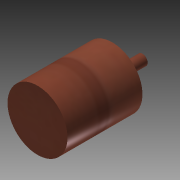
# Autodesk Inventor part: motor
Saved by Autodesk Inventor 2014 (Build 180170000, 170)
## iProperties
Created: 2014-11-30
Part Number: motor
Material: Generic
Document SubType Name: Modeling
Designer: ph1140784
Density: 1 g/cm^3
Appearance: Metal - Ribbed Copper
Mass: 63.6015 g
Surface Area: 92.3628 cm^2
Volume: 63.6015 cm^3
d0: 40.000 mm
d1: 50.000 mm
d2: 0.00 deg
d3: 7.000 mm
d4: 20.000 mm
d5: 0.00 deg
Author: ph1140784
Autodesk Inventor part; units mm, degrees
ref_plane "XZ Plane" through (0, 0, 0) normal (0, 1, 0) x (-1, 0, 0)
ref_plane "XY Plane" through (0, 0, 0) normal (0, 0, 1) x (1, 0, 0)
sketch "Sketch1" plane through (0, 0, 0) normal (0, 1, 0) x (-1, 0, 0)
  circle A0 centre (0, 0) radius 20
  dimension "d0" = 40
  constraints: 1 centre point, 1 coincident
  measures "d0" diameter of A0
extrude "Extrusion1" add sketch "Sketch1" along normal blind 50
sketch "Sketch2" plane through (0, 50, 0) normal (0, 1, 0) x (1, 0, 0)
  circle A0 centre (0, 0) radius 20 projected
  circle A1 centre (0, 0) radius 3.5
  dimension "d3" = 7
  constraints: 1 centre point, 1 coincident
  measures "d3" diameter of A1
extrude "Extrusion2" add sketch "Sketch2" along normal blind 20 contours A1
ref_plane "Work Plane1" through (20, 0, 0) normal (1, 0, 0) x (0, 1, 0)
body "Solid1"
